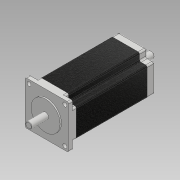
# Autodesk Inventor part: NEMA23, Dual, 113mm Body, 8mm Shaft
Saved by Autodesk Inventor 2018 (Build 220112000, 112)
## iProperties
Created: 2019-05-29
Part Number: NEMA23, Dual, 113mm Body, 8mm Shaft
Material: Generic
Document SubType Name: Modeling
Designer: s.ritter
Density: 1 g/cm^3
Appearance: Default
Author: s.ritter
Autodesk Inventor part; units mm, degrees
ref_plane "YZ Plane" through (0, 0, 0) normal (1, 0, 0) x (0, 1, 0)
sketch "Sketch1" plane through (0, 0, 0) normal (0, 1, 0) x (-1, 0, 0)
  line L0 (28.5, 28.5) -> (-28.5, 28.5)
  line L1 (-28.5, 28.5) -> (-28.5, -28.5)
  line L2 (-28.5, -28.5) -> (28.5, -28.5)
  line L3 (28.5, -28.5) -> (28.5, 28.5)
  line L4 (28.5, 28.5) -> (-28.5, -28.5) construction
  line L5 (-28.5, 28.5) -> (28.5, -28.5) construction
  point P0 (0, 0)
  dimension "d0" = 57
  dimension "d1" = 57
  constraints: 12 end point, 2 midpoint, 2 parallel, 1 horizontal, 1 perpendicular
  measures "d0" distance of L1.end L2.end
  measures "d1" distance of L0.end L1.end
extrude "Extrusion1" add sketch "Sketch1" along normal blind 113
sketch "Sketch2" plane through (0, 113, 0) normal (0, 1, 0) x (1, 0, 0)
  line L0 (-23.5, -23.5) -> (23.5, -23.5) construction
  line L1 (23.5, -23.5) -> (23.5, 23.5) construction
  line L2 (23.5, 23.5) -> (-23.5, 23.5) construction
  line L3 (-23.5, 23.5) -> (-23.5, -23.5) construction
  line L4 (-23.5, -23.5) -> (23.5, 23.5) construction
  line L5 (23.5, -23.5) -> (-23.5, 23.5) construction
  line L6 (-18.5, 18.5) -> (-28.5, 18.5)
  line L7 (-28.5, 18.5) -> (-28.5, 28.5)
  line L8 (-28.5, 28.5) -> (-18.5, 28.5)
  line L9 (-18.5, 28.5) -> (-18.5, 18.5)
  line L10 (-18.5, 18.5) -> (-28.5, 28.5) construction
  line L11 (-28.5, 18.5) -> (-18.5, 28.5) construction
  line L12 (18.5, 18.5) -> (28.5, 18.5)
  line L13 (28.5, 18.5) -> (28.5, 28.5)
  line L14 (28.5, 28.5) -> (18.5, 28.5)
  line L15 (18.5, 28.5) -> (18.5, 18.5)
  line L16 (18.5, 18.5) -> (28.5, 28.5) construction
  line L17 (28.5, 18.5) -> (18.5, 28.5) construction
  line L18 (-28.5, -28.5) -> (28.5, -28.5) construction
  line L19 (18.5, -18.5) -> (28.5, -18.5)
  line L20 (28.5, -18.5) -> (28.5, -28.5)
  line L21 (28.5, -28.5) -> (18.5, -28.5)
  line L22 (18.5, -28.5) -> (18.5, -18.5)
  line L23 (18.5, -18.5) -> (28.5, -28.5) construction
  line L24 (28.5, -18.5) -> (18.5, -28.5) construction
  line L25 (-18.5, -18.5) -> (-28.5, -18.5)
  line L26 (-28.5, -18.5) -> (-28.5, -28.5)
  line L27 (-28.5, -28.5) -> (-18.5, -28.5)
  line L28 (-18.5, -28.5) -> (-18.5, -18.5)
  line L29 (-18.5, -18.5) -> (-28.5, -28.5) construction
  line L30 (-28.5, -18.5) -> (-18.5, -28.5) construction
  point P0 (0, 0)
  dimension "d4" = 47
  dimension "d5" = 47
  constraints: 60 end point, 10 midpoint, 10 parallel, 5 horizontal, 5 perpendicular, 2 point on line, 1 coincident
  measures "d4" distance of L2.end L1.end
  measures "d5" distance of L1.end L0.end
extrude "Extrusion2" cut sketch "Sketch2" against normal blind 108
fillet "Fillet1" radius 2 16 edges at (28.5, 59, 18.5) (18.5, 59, 18.5) (18.5, 59, 28.5) (-18.5, 59, 28.5) (-18.5, 59, 18.5) (-28.5, 59, 18.5) (-28.5, 59, -18.5) (-18.5, 59, -18.5) (-18.5, 59, -28.5) (18.5, 59, -28.5) (18.5, 59, -18.5) (28.5, 59, -18.5) (-28.5, 2.5, -28.5) (28.5, 2.5, -28.5) (28.5, 2.5, 28.5) (-28.5, 2.5, 28.5)
fillet "Fillet2" radius 2 24 edges at (-17.9142, 113, -27.9142) (-18.5, 113, -23.5) (-19.0858, 113, -19.0858) (-23.5, 113, -18.5) (-27.9142, 113, -17.9142) (-28.5, 113, 0) (-27.9142, 113, 17.9142) (-23.5, 113, 18.5) (-19.0858, 113, 19.0858) (-18.5, 113, 23.5) (-17.9142, 113, 27.9142) (0, 113, 28.5) (17.9142, 113, 27.9142) (18.5, 113, 23.5) (19.0858, 113, 19.0858) (23.5, 113, 18.5) (27.9142, 113, 17.9142) (28.5, 113, 0) (27.9142, 113, -17.9142) (23.5, 113, -18.5) (19.0858, 113, -19.0858) (18.5, 113, -23.5) (17.9142, 113, -27.9142) (0, 113, -28.5)
sketch "Sketch3" plane through (0, 0, 0) normal (0, -1, 0) x (1, 0, 0)
  line L0 (23.5, -23.5) -> (-23.5, -23.5) construction
  line L1 (-23.5, -23.5) -> (-23.5, 23.5) construction
  line L2 (-23.5, 23.5) -> (23.5, 23.5) construction
  line L3 (23.5, 23.5) -> (23.5, -23.5) construction
  line L4 (23.5, -23.5) -> (-23.5, 23.5) construction
  line L5 (-23.5, -23.5) -> (23.5, 23.5) construction
  point P0 (0, 0)
  dimension "d10" = 47
  dimension "d11" = 47
  constraints: 12 end point, 2 midpoint, 2 parallel, 1 horizontal, 1 perpendicular
  measures "d10" distance of L1.end L2.end
  measures "d11" distance of L0.end L1.end
hole "Hole1" at (23.5, 0, -23.5) at (-23.5, 0, 23.5) at (-23.5, 0, -23.5) at (23.5, 0, 23.5) direction (0, 1, 0) diameter 5.3 end through all clearance for "Socket Head Cap Screw" size "M5" standard "Ansi Metric M Profile"
sketch "Sketch4" plane through (0, 0, 0) normal (0, -1, 0) x (1, 0, 0)
  circle A0 centre (0, 0) radius 19.05
  dimension "d19" = 38.1
  constraints: 1 centre point, 1 coincident
  measures "d19" diameter of A0
extrude "Extrusion3" add sketch "Sketch4" along normal blind 1.8
sketch "Sketch5" plane through (0, -1.8, 0) normal (0, -1, 0) x (1, 0, 0)
  circle A0 centre (0, 0) radius 4
  dimension "d22" = 8
  constraints: 1 centre point, 1 coincident
  measures "d22" diameter of A0
extrude "Extrusion4" add sketch "Sketch5" along normal blind 24 from surface at -1.8
sketch "Sketch6" plane through (0, -24, 0) normal (0, -1, 0) x (1, 0, 0)
  line L0 (28.5, -28.5) -> (-28.5, -28.5)
  line L1 (-28.5, -28.5) -> (-28.5, -3.5)
  line L2 (-28.5, -3.5) -> (28.5, -3.5)
  line L3 (28.5, -3.5) -> (28.5, -28.5)
  line L4 (28.5, 26.5) -> (28.5, -26.5) projected
  line L5 (-28.5, -26.5) -> (-28.5, 26.5) projected
  line L6 (26.5, -28.5) -> (-26.5, -28.5) projected
  point P0 (0, 0)
  dimension "d25" = 3.5
  constraints: 8 end point, 3 collinear, 2 parallel, 1 horizontal, 1 perpendicular
  measures "d25" distance from line of L2 point (0, 0)
extrude "Extrusion5" cut sketch "Sketch6" against normal blind 20
chamfer "Chamfer1" distance 0.5 angle 45 3 edges at (3.4457, -24, -2.0315) (-2.0315, -24, 3.4457) (0, -24, -3.5)
ref_plane "Work Plane1" through (0, 10, 0) normal (0, -1, 0) x (1, 0, 0)
ref_plane "Work Plane2" through (0, 103, 0) normal (0, 1, 0) x (1, 0, 0)
split_face "Split1"
split_face "Split2"
sketch "Sketch7" plane through (0, 113, 0) normal (0, 1, 0) x (1, 0, 0)
  arc A0 (-1.9365, 3.5) -> (1.9365, 3.5) centre (0, 0) ccw projected
  line L0 (-1.9365, 3.5) -> (1.9365, 3.5) projected
  circle A1 centre (0, 0) radius 4 projected
extrude "Extrusion6" add sketch "Sketch7" along normal blind 24 contours L0 A0
extrude "Extrusion7" add sketch "Sketch7" along normal blind 4 contours A1 L0
chamfer "Chamfer2" distance 0.5 angle 45 2 edges at (0, 137, 4) (0, 137, -3.5)
body "Solid1"
